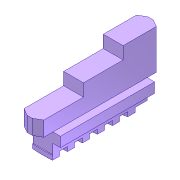
# Autodesk Inventor part: Jaw2
Saved by Autodesk Inventor 2016 (Build 200138000, 138)
## iProperties
Created: 2011-02-15
Part Number: Jaw2
Document SubType Name: Modeling
Designer: nguyenducthang
Density: 1 g/cm^3
Mass: 0.958199 g
Surface Area: 8.72012 cm^2
Volume: 0.958199 cm^3
Material: Generic
Appearance: Violet
Author: nguyenducthang
Autodesk Inventor part; units mm, degrees
ref_plane "YZ Plane" through (0, 0, 0) normal (1, 0, 0) x (0, 1, 0)
ref_plane "XZ Plane" through (0, 0, 0) normal (0, 1, 0) x (-1, 0, 0)
ref_plane "XY Plane" through (0, 0, 0) normal (0, 0, 1) x (1, 0, 0)
sketch "Sketch10" plane through (0, 0, 0) normal (0, 0, 1) x (1, 0, 0)
  line L0 (0, 0) -> (-2, 0)
  line L1 (-2, 0) -> (-2, 2)
  line L2 (-2, 2) -> (-3.5, 2)
  line L3 (-3.5, 2) -> (-3.5, 4)
  line L4 (-3.5, 4) -> (-2, 4)
  line L5 (-2, 4) -> (-2, 12)
  line L6 (-2, 12) -> (0, 12)
  line L7 (0, 12) -> (0, 0) construction
  line L8 (0, 0) -> (2, 0)
  line L9 (2, 0) -> (2, 2)
  line L10 (2, 2) -> (3.5, 2)
  line L11 (3.5, 2) -> (3.5, 4)
  line L12 (3.5, 4) -> (2, 4)
  line L13 (2, 4) -> (2, 12)
  line L14 (2, 12) -> (0, 12)
  dimension "d51" = 2
  dimension "d52" = 3.5
  dimension "d53" = 2
  dimension "d54" = 2
  dimension "d55" = 2
  dimension "d56" = 8
  constraints: 30 end point, 6 symmetric about line, 5 parallel, 1 collinear, 1 horizontal, 1 perpendicular, 1 other
  measures "d51" distance of L0.start L0.end
  measures "d52" distance between parallel lines of L3 L7
  measures "d53" distance between parallel lines of L5 L7
  measures "d54" distance of L0.end L1.end
  measures "d55" distance of L2.end L3.end
  measures "d56" distance of L4.end L5.end
extrude "Extrusion8" add sketch "Sketch10" along normal blind 25
sketch "Sketch11" plane through (-2, 12, 0) normal (0, 1, 0) x (1, 0, 0)
  line L0 (0, -25) -> (4, -25) projected
  line L1 (0, 0) -> (4, 0) projected
  line L2 (-1.5, 0) -> (-1.5, -25) projected
  line L3 (5.5, 0) -> (5.5, -25) projected
  line L4 (2, 0) -> (-1.5, -2.0207)
  line L5 (2, 0) -> (5.5, -2.0207)
  line L6 (-1.5, -2.0207) -> (-1.5, 0)
  line L7 (-1.5, 0) -> (5.5, 0)
  line L8 (5.5, -2.0207) -> (5.5, 0)
  line L9 (2, -25) -> (-1.5, -22.9793)
  line L10 (2, -25) -> (5.5, -22.9793)
  line L11 (-1.5, -22.9793) -> (-1.5, -25)
  line L12 (-1.5, -25) -> (5.5, -25)
  line L13 (5.5, -25) -> (5.5, -22.9793)
  dimension "d59" = 30
  dimension "d60" = 30
  constraints: 20 end point, 5 collinear, 4 point on line, 2 midpoint, 2 parallel, 1 perpendicular
  measures "d59" angle of L1 L5
  measures "d60" angle of L1 L4
extrude "Extrusion9" cut sketch "Sketch11" against normal through all contours L12 L2 L9 L0 | L10 L3 L12 L0 | L2 L7 L1 L4 | L5 L1 L7 L3
sketch "Sketch12" plane through (-2, 12, 23.8453) normal (0, 1, 0) x (1, 0, 0)
  line L0 (0, 22.6906) -> (0, 0) projected
  line L1 (0, 0) -> (2, -1.1547) projected
  line L2 (2, -1.1547) -> (4, 0) projected
  line L3 (4, 22.6906) -> (4, 0) projected
  line L4 (0, 8) -> (4, 8)
  dimension "d63" = 8
  constraints: 2 end point, 2 point on line, 1 perpendicular
  measures "d63" distance from line of L4 L0.end
extrude "Extrusion10" cut sketch "Sketch12" against normal blind 5
sketch "Sketch13" plane through (-2, 12, 15.8453) normal (0, 1, 0) x (1, 0, 0)
  line L0 (0, 0) -> (4, 0) projected
  line L1 (4, 14.6906) -> (4, 0) projected
  line L2 (0, 14.6906) -> (0, 0) projected
  line L3 (0, 8) -> (4, 8)
  dimension "d66" = 8
  constraints: 2 end point, 2 point on line, 1 perpendicular
  measures "d66" distance between parallel lines of L3 L0
extrude "Extrusion11" cut sketch "Sketch13" against normal blind 2.5
sketch "Sketch15" plane through (2, 0, 1.1547) normal (0, -1, 0) x (1, 0, 0)
  line L0 (-2, -1.1547) -> (0, 0) projected
  line L1 (0, 0) -> (0, 22.6906) projected
  line L2 (0, 22.6906) -> (-2, 23.8453) projected
  line L3 (-2, 23.8453) -> (-4, 22.6906) projected
  line L4 (-4, 0) -> (-2, -1.1547) projected
  line L5 (-5.5, 0.866) -> (-5.5, 21.8246) projected
  line L6 (1.5, 0.866) -> (1.5, 21.8246) projected
  line L7 (-5.5, 20.8453) -> (1.5, 20.8453)
  line L8 (1.5, 20.8453) -> (1.5, 21.8246)
  line L9 (1.5, 21.8246) -> (-2, 23.8453)
  line L10 (-2, 23.8453) -> (-5.5, 21.8246)
  line L11 (-5.5, 21.8246) -> (-5.5, 20.8453)
  line L12 (-2, -1.1547) -> (-5.5, 0.866)
  line L13 (-5.5, 0.866) -> (-5.5, 1.8453)
  line L14 (-5.5, 1.8453) -> (1.5, 1.8453)
  line L15 (1.5, 1.8453) -> (1.5, 0.866)
  line L16 (1.5, 0.866) -> (-2, -1.1547)
  dimension "d72" = 3
  dimension "d73" = 3
  constraints: 20 end point, 7 collinear, 4 point on line, 2 perpendicular
  measures "d72" distance from line of L7 L2.end
  measures "d73" distance from line of L14 L0.start
extrude "Extrusion13" cut sketch "Sketch15" against normal up to surface (4 mm away) contours L4 L12 L5 L14 L1 L0 | L1 L14 L6 L16 | L7 L5 L10 L3 L2 L1 | L1 L9 L6 L7
sketch "Sketch16" plane through (-2, 0, 3) normal (0, -1, 0) x (1, 0, 0)
  line L0 (4, 0) -> (4, 19) projected
  line L1 (0, 0) -> (0, 19) projected
  arc A0 (4, 2.4443) -> (0, 2.4443) centre (2, -3) ccw
  arc A1 (4, 3.9166) -> (0, 3.9166) centre (2, -3) ccw
  arc A2 (4, 5.5697) -> (0, 5.5697) centre (2, -3) ccw
  arc A3 (4, 7.002) -> (0, 7.002) centre (2, -3) ccw
  arc A4 (4, 8.6293) -> (0, 8.6293) centre (2, -3) ccw
  arc A5 (4, 10.0476) -> (0, 10.0476) centre (2, -3) ccw
  arc A6 (4, 11.6642) -> (0, 11.6642) centre (2, -3) ccw
  arc A7 (4, 13.0761) -> (0, 13.0761) centre (2, -3) ccw
  arc A8 (4, 16.0955) -> (0, 16.0955) centre (2, -3) ccw
  line L2 (0, 2.4443) -> (0, 3.9166)
  line L3 (0, 5.5697) -> (0, 7.002)
  line L4 (0, 8.6293) -> (0, 10.0476)
  line L5 (0, 11.6642) -> (0, 13.0761)
  line L6 (4, 2.4443) -> (4, 3.9166)
  line L7 (4, 5.5697) -> (4, 7.002)
  line L8 (4, 8.6293) -> (4, 10.0476)
  line L9 (4, 11.6642) -> (4, 13.0761)
  arc A9 (4, 14.6873) -> (0, 14.6873) centre (2, -3) ccw
  arc A10 (4, 17.7036) -> (0, 17.7036) centre (2, -3) ccw
  arc A11 (4, 19.1097) -> (0, 19.1097) centre (2, -3) ccw
  line L10 (0, 14.6873) -> (0, 16.0955)
  line L11 (0, 17.7036) -> (0, 19.1097)
  line L12 (4, 17.7036) -> (4, 19.1097)
  line L13 (4, 16.0955) -> (4, 14.6873)
  dimension "d76" = 11.6
  dimension "d79" = 1.4
  dimension "d81" = 1.4
  dimension "d83" = 1.4
  dimension "d85" = 1.4
  dimension "d87" = 1.4
  dimension "d89" = 1.4
  dimension "d92" = 3
  dimension "d93" = 3
  dimension "d94" = 3
  dimension "d95" = 3
  dimension "d96" = 3
  constraints: 24 end point, 24 point on circle, 12 centre point, 12 vertical, 1 coincident, 26 other
  measures "d76" diameter of A0
  measures "d79" radial gap between concentric circles of A1 A0
  measures "d81" radial gap between concentric circles of A3 A2
  measures "d83" radial gap between concentric circles of A5 A4
  measures "d85" radial gap between concentric circles of A7 A6
  measures "d87" radial gap between concentric circles of A8 A9
  measures "d89" radial gap between concentric circles of A11 A10
  measures "d92" radial gap between concentric circles of A2 A0
  measures "d93" radial gap between concentric circles of A4 A2
  measures "d94" radial gap between concentric circles of A6 A4
  measures "d95" radial gap between concentric circles of A9 A6
  measures "d96" radial gap between concentric circles of A10 A9
extrude "Extrusion14" add sketch "Sketch16" along normal blind 0.9 contours A0 L1 A1 L0 | A2 L1 A3 L0 | A4 L1 A5 L0 | A6 L1 A7 L0 | A9 L1 A8 L0 | A10 L1 L11 A11 L12 L0
fillet "Fillet1" radius 0.02 12 edges at (0, -0.9, 22.2) (0, -0.9, 20.8) (0, -0.9, 19.2) (0, -0.9, 17.8) (0, -0.9, 16.2) (0, -0.9, 14.8) (0, -0.9, 13.2) (0, -0.9, 11.8) (0, -0.9, 10.2) (0, -0.9, 8.8) (0, -0.9, 7.2) (0, -0.9, 5.8)
sketch "Sketch18" plane through (-2, 4, 3) normal (0, -1, 0) x (1, 0, 0)
  line L0 (2, -3) -> (0, -1.8453) projected
  line L1 (4, -1.8453) -> (2, -3) projected
  line L2 (0, 19) -> (0, 20.8453) projected
  line L3 (0, 19) -> (4, 19) projected
  line L4 (4, 19) -> (4, 20.8453) projected
  line L5 (2, 22) -> (4, 20.8453) projected
  line L6 (0, 20.8453) -> (2, 22) projected
  line L7 (1.4804, -2.7) -> (2.5196, -2.7)
  line L8 (2.5196, 21.7) -> (1.4804, 21.7)
  dimension "d103" = 0.3
  dimension "d104" = 0.3
  constraints: 4 end point, 4 point on line, 1 parallel, 1 perpendicular
  measures "d103" distance from line of L7 L0.start
  measures "d104" distance from line of L8 L5.start
extrude "Extrusion16" cut sketch "Sketch18" against normal through all contours L0 L7 L1 | L6 L5 L8
body "Solid1"
